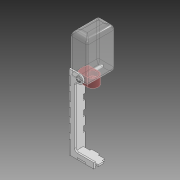
# Autodesk Inventor part: Узел_наклона
Saved by Autodesk Inventor 2022 (Build 260153000, 153)
## iProperties
Created: 2025-01-31
Part Number: Узел_наклона
Material: Типовые
Document SubType Name: Modeling
Designer: Ivan
Density: 1 g/cm^3
Appearance: По умолчанию
Author: Ivan
Autodesk Inventor part; units mm, degrees
ref_plane "YZ Plane" through (0, 0, 0) normal (1, 0, 0) x (0, 1, 0)
ref_plane "XZ Plane" through (0, 0, 0) normal (0, 1, 0) x (-1, 0, 0)
ref_plane "XY Plane" through (0, 0, 0) normal (0, 0, 1) x (1, 0, 0)
sketch "Эскиз1" plane through (0, 0, 0) normal (0, 0, 1) x (1, 0, 0)
  line L0 (0, 0) -> (0, 30.9191)
  line L1 (5, 0) -> (5, 15)
  line L2 (5, 15) -> (15.25, 15)
  line L3 (15.25, 15) -> (15.25, 31)
  line L4 (15.25, 31) -> (40, 31)
  line L5 (40, 31) -> (40, 0)
  line L6 (40, 0) -> (5, 0)
  dimension "d0" = 10
  dimension "d1" = 30.5
  dimension "d2" = 16
  dimension "d3" = 15
  dimension "d4" = 80
  constraints: 14 end point, 5 perpendicular, 2 vertical, 1 point on line
  measures "d0" diameter of L1 L0
  measures "d1" diameter of L3 L0
  measures "d2" distance of L2.end L3.end
  measures "d3" distance of L1.start L1.end
  measures "d4" diameter of L5 L0
revolve "Вращение1" add sketch "Эскиз1" angle 360 about axis through (0, 0, 0) along (0, 1, 0)
sketch "Эскиз2" plane through (0, 15, 0) normal (0, 1, 0) x (1, 0, 0)
  ellipse E0 centre (0, 0) end of major axis (0, 14) minor radius 8
  dimension "d6" = 14
  dimension "d7" = 8
  constraints: 1 coincident, 2 other
extrude "Выдавливание1" cut sketch "Эскиз2" against normal through all
sketch "Эскиз3" plane through (0, 0, 0) normal (0, 0, 1) x (1, 0, 0)
  circle A0 centre (-25, 15.5) radius 4.1
  line L0 (-40, 31) -> (-40, 0) construction
  point P0 (0, 0)
  point P1 (-40, 15.5)
  dimension "d10" = 8.2
  dimension "d11" = 25
  constraints: 1 centre point, 1 horizontal alignment, 1 midpoint
  measures "d10" diameter of A0
  measures "d11" horizontal distance of point (0, 0) A0.centre
extrude "Выдавливание2" cut sketch "Эскиз3" along normal through all both and the other way through all
sketch "Эскиз4" plane through (0, 31, 0) normal (0, 1, 0) x (1, 0, 0)
  line L0 (45.6039, -20) -> (-45.6039, -20)
  line L1 (-45.6039, -20) -> (-45.6039, 20)
  line L2 (-45.6039, 20) -> (45.6039, 20)
  line L3 (45.6039, 20) -> (45.6039, -20)
  ellipse E0 centre (0, 0) end of major axis (0, 14) minor radius 8 projected
  line L4 (45.6039, -20) -> (-45.6039, 20) construction
  line L5 (-45.6039, -20) -> (45.6039, 20) construction
  line L6 (-60.9114, -53.5893) -> (60.9114, -53.5893)
  line L7 (60.9114, -53.5893) -> (60.9114, 53.5893)
  line L8 (60.9114, 53.5893) -> (-60.9114, 53.5893)
  line L9 (-60.9114, 53.5893) -> (-60.9114, -53.5893)
  line L10 (-60.9114, -53.5893) -> (60.9114, 53.5893) construction
  line L11 (60.9114, -53.5893) -> (-60.9114, 53.5893) construction
  circle A0 centre (0, 0) radius 20
  point P0 (0, 20)
  point P1 (0, -20)
  dimension "d14" = 40
  constraints: 24 end point, 4 midpoint, 4 parallel, 2 horizontal, 2 perpendicular, 1 centre point, 1 coincident, 1 tangent, 1 other
  measures "d14" distance of L0.end L1.end
extrude "Выдавливание3" cut sketch "Эскиз4" against normal through all contours L0 A0 L2 L3 | L9 L8 L7 L6
fillet "Сопряжение1" radius 5 2 edges at (-34.641, 15.5, 20) (-34.641, 15.5, -20)
sketch "Эскиз5" plane through (0, 0, 0) normal (1, 0, 0) x (0, 1, 0)
  line L0 (0, 0) -> (47.7229, 0) construction
  line L1 (31, 17.1429) -> (31, -17.1429) projected
  line L2 (10.8203, 0) -> (31, 0)
  line L3 (31, 0) -> (31, -15.8105)
  line L4 (31, -15.8105) -> (10.8203, -15.8105)
  line L5 (10.8203, -15.8105) -> (10.8203, 0)
  constraints: 10 end point, 2 horizontal, 2 parallel, 2 point on line, 1 perpendicular
revolve "Вращение2" add sketch "Эскиз5" angle 360 about axis through (0, 0, 0) along (0, 1, 0) separate body
sketch "Эскиз6" plane through (0, 31, 0) normal (0, 1, 0) x (1, 0, 0)
  line L0 (25, 50) -> (-25, 50)
  line L1 (-30, 45) -> (-30, -45)
  line L2 (-25, -50) -> (25, -50)
  line L3 (30, -45) -> (30, 45)
  line L4 (30, 50) -> (-30, -50) construction
  line L5 (-30, 50) -> (30, -50) construction
  arc A0 (25, -50) -> (30, -45) centre (25, -45) ccw
  arc A1 (-30, -45) -> (-25, -50) centre (-25, -45) ccw
  arc A2 (-25, 50) -> (-30, 45) centre (-25, 45) ccw
  arc A3 (30, 45) -> (25, 50) centre (25, 45) ccw
  point P0 (0, 0)
  dimension "d19" = 100
  dimension "d20" = 60
  dimension "d21" = 5
  constraints: 12 end point, 8 point on circle, 8 point on line, 8 tangent, 4 centre point, 3 equal radius, 2 midpoint, 2 parallel, 1 horizontal, 1 perpendicular
  measures "d19" distance of L5.start L4.end
  measures "d20" distance of L4.end L5.end
  measures "d21" radius of A0
extrude "Выдавливание4" add sketch "Эскиз6" along normal blind 150 bodies 2
fillet "Сопряжение2" radius 20 8 edges at (-28.5355, 181, -48.5355) (-30, 181, 0) (-28.5355, 181, 48.5355) (0, 181, 50) (28.5355, 181, 48.5355) (30, 181, 0) (28.5355, 181, -48.5355) (0, 181, -50)
fillet "Сопряжение3" radius 10 8 edges at (-28.5355, 31, 48.5355) (0, 31, 50) (28.5355, 31, 48.5355) (30, 31, 0) (28.5355, 31, -48.5355) (0, 31, -50) (-28.5355, 31, -48.5355) (-30, 31, 0)
sketch "Эскиз7" plane through (0, 0, 0) normal (0, 0, 1) x (1, 0, 0)
  circle A0 centre (-25, 15.5) radius 4.1 projected
  point P0 (0, 0)
extrude "Выдавливание5" add sketch "Эскиз7" along normal blind 26 and the other way blind 60 separate body
sketch "Эскиз8" plane through (0, 0, 20) normal (0, 0, 1) x (1, 0, 0)
  circle A0 centre (-25, 15.5) radius 4.1 construction
  circle A1 centre (-25, 15.5) radius 4.1 construction
  circle A2 centre (-25, 15.5) radius 15.5
  line L0 (0, 31) -> (-31.6228, 31) construction
  line L1 (-10.4348, 20.8013) -> (30, -90.2923)
  line L2 (30, -90.2923) -> (30, -239)
  line L3 (-15.8105, 10.8203) -> (15.8105, 10.8203) construction
  line L4 (30, -239) -> (-60, -239)
  line L5 (-60, -239) -> (-60, 31)
  line L6 (-60, 31) -> (-25, 31)
  arc A3 (-30, 41) -> (-20, 31) centre (-20, 41) ccw projected
  line L7 (0, 0) -> (0, -302.6843) construction
  line L8 (-40, 31) -> (-40, 0) construction
  circle A4 centre (-25, 15.5) radius 10.9
  dimension "d30" = 270
  dimension "d31" = 20
  dimension "d32" = 20
  dimension "d33" = 90
  dimension "d34" = 21.8
  constraints: 12 end point, 3 perpendicular, 3 point on circle, 3 tangent, 2 centre point, 2 coincident, 1 horizontal, 1 vertical
  measures "d30" distance between parallel lines of L4 L6
  measures "d31" angle of L2 L1
  measures "d32" distance between parallel lines of L8 L5
  measures "d33" distance between parallel lines of L2 L5
  measures "d34" diameter of A4
extrude "Выдавливание6" add sketch "Эскиз8" along normal blind 6 separate body
sketch "Эскиз9" plane through (0, 0, 20) normal (0, 0, 1) x (1, 0, 0)
  circle A0 centre (-25, 15.5) radius 10.9 projected
  circle A1 centre (-25, 15.5) radius 4.1 projected
  point P0 (0, 0)
extrude "Выдавливание7" add sketch "Эскиз9" along normal blind 7 separate body
sketch "Эскиз10" plane through (-60, -239, 20) normal (-1, 0, 0) x (0, 0, 1)
  line L0 (6, 270) -> (-46, 270)
  line L1 (-46, 270) -> (-46, 0)
  line L2 (-46, 0) -> (6, 0)
  line L3 (6, 0) -> (6, 270)
  line L4 (-40, 270) -> (-40, 239) construction
  point P0 (-20, 239)
  dimension "d39" = 6
  constraints: 8 end point, 2 parallel, 1 horizontal, 1 perpendicular, 1 point on line
  measures "d39" distance between parallel lines of L1 L4
extrude "Выдавливание8" add sketch "Эскиз10" against normal blind 6 separate body
sketch "Эскиз11" plane through (-60, -239, 20) normal (0, -1, 0) x (1, 0, 0)
  line L0 (0, 6) -> (90, 6) projected
  line L1 (0, 6) -> (90, 6)
  line L2 (90, 6) -> (90, -46)
  line L3 (90, -46) -> (0, -46)
  line L4 (0, -46) -> (0, 6)
  line L5 (90, 0) -> (90, 6) projected
  line L6 (0, -46) -> (6, -46) projected
  point P0 (60, -20)
  constraints: 8 end point, 2 collinear, 2 parallel, 1 horizontal, 1 perpendicular
extrude "Выдавливание9" add sketch "Эскиз11" against normal blind 6 separate body
sketch "Эскиз12" plane through (-60, -239, 20) normal (-1, 0, 0) x (0, 0, 1)
  line L0 (-20, 239) -> (-20, 10.9172) construction
  line L1 (-46, 0) -> (-46, 270) construction
  line L2 (-46, 135) -> (6, 135) construction
  line L3 (6, 270) -> (6, 0) construction
  line L4 (6, 0) -> (-46, 0) construction
  line L5 (-30, 0) -> (-10, 0)
  line L6 (-10, 0) -> (-10, 6)
  line L7 (-10, 6) -> (-30, 6)
  line L8 (-30, 6) -> (-30, 0)
  line L9 (6, 120) -> (0, 120)
  line L10 (0, 120) -> (0, 100)
  line L11 (0, 100) -> (6, 100)
  line L12 (6, 100) -> (6, 120)
  line L13 (6, 70) -> (0, 70)
  line L14 (0, 70) -> (0, 50)
  line L15 (0, 50) -> (6, 50)
  line L16 (6, 50) -> (6, 70)
  line L17 (6, 150) -> (0, 150)
  line L18 (0, 150) -> (0, 170)
  line L19 (0, 170) -> (6, 170)
  line L20 (6, 170) -> (6, 150)
  line L21 (6, 200) -> (0, 200)
  line L22 (0, 200) -> (0, 220)
  line L23 (0, 220) -> (6, 220)
  line L24 (6, 220) -> (6, 200)
  line L25 (-46, 120) -> (-40, 120)
  line L26 (-40, 120) -> (-40, 100)
  line L27 (-40, 100) -> (-46, 100)
  line L28 (-46, 100) -> (-46, 120)
  line L29 (-46, 70) -> (-40, 70)
  line L30 (-40, 70) -> (-40, 50)
  line L31 (-40, 50) -> (-46, 50)
  line L32 (-46, 50) -> (-46, 70)
  line L33 (-40, 150) -> (-40, 170)
  line L34 (-40, 170) -> (-46, 170)
  line L35 (-46, 170) -> (-46, 150)
  line L36 (-46, 200) -> (-40, 200)
  line L37 (-40, 200) -> (-40, 220)
  line L38 (-40, 220) -> (-46, 220)
  line L39 (-46, 220) -> (-46, 200)
  line L40 (-46, 150) -> (-40, 150)
  line L41 (6, 148.7077) -> (6, 259.8013) projected
  line L42 (6, 250) -> (0, 250)
  line L43 (0, 250) -> (0, 270)
  line L44 (0, 270) -> (6, 270)
  line L45 (6, 270) -> (6, 250)
  line L46 (0, 270) -> (6, 270) projected
  line L47 (-46, 250) -> (-40, 250)
  line L48 (-40, 250) -> (-40, 270)
  line L49 (-40, 270) -> (-46, 270)
  line L50 (-46, 270) -> (-46, 250)
  line L51 (-40, 270) -> (-46, 270)
  point P0 (-46, 259.8013)
  dimension "d44" = 6
  dimension "d45" = 20
  dimension "d46" = 20
  dimension "d47" = 6
  dimension "d48" = 15
  dimension "d49" = 30
  constraints: 94 end point, 31 symmetric about line, 8 parallel, 8 point on line, 4 horizontal, 4 perpendicular, 3 equal length, 2 midpoint, 1 collinear, 1 vertical, 1 other
  measures "d44" distance of L5.end L6.end
  measures "d45" distance of L6.end L7.end
  measures "d46" distance of L9.end L10.end
  measures "d47" distance of L9.start L9.end
  measures "d48" distance between parallel lines of L2 L9
  measures "d49" distance between parallel lines of L13 L11
extrude "Выдавливание10" cut sketch "Эскиз12" against normal through all bodies 6
sketch "Эскиз13" plane through (0, 0, 26) normal (0, 0, 1) x (1, 0, 0)
  line L0 (-60, -19) -> (-54, -19) projected
  line L1 (-54, -89) -> (-54, -119) projected
  line L2 (-60, -239) -> (-60, -189) projected
  line L3 (-60, -69) -> (-54, -69) projected
  line L4 (-54, -39) -> (-54, -69)
  line L5 (-54, -39) -> (-60, -39) projected
  line L6 (-60, -69) -> (-60, -39) projected
  line L7 (-54, -89) -> (-60, -89) projected
  line L8 (-60, -119) -> (-60, -89)
  line L9 (-60, -119) -> (-54, -119) projected
  line L10 (-54, -89) -> (-54, -119) projected
  line L11 (-60, -169) -> (-54, -169) projected
  line L12 (-54, -139) -> (-54, -169) projected
  line L13 (-54, -139) -> (-60, -139) projected
  line L14 (-60, -169) -> (-60, -139)
  line L15 (-54, -189) -> (-60, -189) projected
  line L16 (-60, -239) -> (-60, -189) projected
  line L17 (-60, -239) -> (-54, -239) projected
  line L18 (-54, -189) -> (-54, -239)
  line L19 (-60, -239) -> (30, -239) construction
  line L20 (-30, -239) -> (0, -239)
  line L21 (0, -239) -> (0, -233)
  line L22 (0, -233) -> (-30, -233)
  line L23 (-30, -233) -> (-30, -239)
  line L24 (-60, -119) -> (-54, -119) projected
  line L25 (-54, -89) -> (-60, -89) projected
  line L26 (-60, -119) -> (-60, -89) projected
  line L27 (-54, -139) -> (-60, -139) projected
  line L28 (-60, -169) -> (-60, -139) projected
  line L29 (-60, -169) -> (-54, -169) projected
  line L30 (-54, -139) -> (-54, -169) projected
  line L31 (-54, 11) -> (-54, -19)
  line L32 (-54, 11) -> (-60, 11) projected
  line L33 (-60, -19) -> (-60, 11) projected
  line L34 (-54, -39) -> (-60, -39) projected
  line L35 (-60, -69) -> (-60, -39) projected
  line L36 (-60, -69) -> (-54, -69) projected
  line L37 (-54, -39) -> (-54, -69) projected
  line L38 (-54, -189) -> (-60, -189) projected
  line L39 (-60, -239) -> (-54, -239) projected
  line L40 (-54, -189) -> (-54, -239) projected
  point P0 (0, 0)
  point P1 (-15, -239)
  point P2 (-15, -239)
  dimension "d52" = 30
  constraints: 18 end point, 2 midpoint, 2 parallel, 2 perpendicular, 1 coincident, 1 horizontal, 1 point on line
  measures "d52" distance of L21.end L22.end
extrude "Выдавливание11" cut sketch "Эскиз13" against normal through all bodies 4
sketch "Эскиз14" plane through (-60, -239, 20) normal (0, -1, 0) x (1, 0, 0)
  line L0 (90, -46) -> (0, -46) construction
  line L1 (45, -46) -> (45, 5.2273) construction
  line L2 (45.9, 7) -> (24.1, 7) construction
  line L3 (60, -20) -> (-12.0098, -20) construction
  line L4 (0, -10) -> (6, -10) projected
  line L5 (6, 6) -> (6, -10) projected
  line L6 (0, 6) -> (6, 6) projected
  line L7 (0, -10) -> (0, 6) projected
  line L8 (6, -30) -> (0, -30) projected
  line L9 (0, -46) -> (0, -30) projected
  line L10 (0, -46) -> (6, -46) projected
  line L11 (6, -30) -> (6, -46) projected
  line L12 (6, 6) -> (6, 0) projected
  line L13 (60, 0) -> (90, 0) projected
  line L14 (30, 0) -> (30, 6) projected
  line L15 (6, 6) -> (30, 6) projected
  line L16 (60, 6) -> (60, 0) projected
  line L17 (60, 0) -> (90, 0) projected
  line L18 (90, 0) -> (90, 6) projected
  line L19 (60, 6) -> (90, 6)
  line L20 (90, -10) -> (84, -10)
  line L21 (84, 6) -> (84, -10)
  line L22 (90, 6) -> (84, 6)
  line L23 (90, -10) -> (90, 6)
  line L24 (84, -30) -> (90, -30)
  line L25 (90, -46) -> (90, -30)
  line L26 (90, -46) -> (84, -46)
  line L27 (84, -30) -> (84, -46)
  line L28 (84, 6) -> (84, 0)
  line L29 (45.9, -47) -> (24.1, -47) construction
  line L30 (0, -46) -> (6, -46)
  line L31 (6, -46) -> (6, -40)
  line L32 (6, -40) -> (30, -40)
  line L33 (30, -40) -> (30, -46)
  line L34 (6, -46) -> (30, -46)
  line L35 (60, -46) -> (60, -40)
  line L36 (60, -40) -> (90, -40)
  line L37 (90, -40) -> (90, -46)
  line L38 (60, -46) -> (90, -46)
  line L39 (84, -46) -> (84, -40)
  line L40 (90, -46) -> (84, -46)
  line L41 (6, 0) -> (30, 0)
  line L42 (60, 6) -> (60, 0) projected
  line L43 (90, 0) -> (90, 6) projected
  line L44 (60, 6) -> (90, 6) projected
  point P0 (102.0098, -20)
  point P1 (45, -45.2273)
  constraints: 50 end point, 25 symmetric about line, 1 horizontal, 1 midpoint, 1 perpendicular
extrude "Выдавливание12" cut sketch "Эскиз14" against normal through all bodies 7
sketch "Эскиз15" plane through (0, 0, 26) normal (0, 0, 1) x (1, 0, 0)
  circle A0 centre (-25, 15.5) radius 4.1 projected
  circle A1 centre (-25, 15.5) radius 4.1 projected
  arc A2 (-10.4348, 20.8013) -> (-25, 31) centre (-25, 15.5) ccw projected
  circle A3 centre (-25, 15.5) radius 15.5
  line L0 (-31.6228, 0) -> (0, 0) projected
  line L1 (-40, -219) -> (30, -219)
  line L2 (30, -239) -> (30, -90.2923) projected
  line L3 (30, -90.2923) -> (-10.4348, 20.8013) projected
  line L4 (0, -239) -> (30, -239) projected
  line L5 (-25, 0) -> (-40, 0)
  line L6 (-40, 0) -> (-40, -219)
  point P0 (-10.4348, 20.8013)
  dimension "d59" = 20
  dimension "d63" = 70
  constraints: 6 end point, 2 horizontal, 2 point on circle, 2 point on line, 1 centre point, 1 coincident, 1 perpendicular
  measures "d59" distance between parallel lines of L4 L1
  measures "d63" distance between parallel lines of L6 L2
extrude "Выдавливание13" cut sketch "Эскиз15" against normal through all contours L3 L0 A3 | L3 L2 L1 L6 L5 L0 bodies 4
fillet "Сопряжение4" radius 10 3 edges at (-25, 0, 23) (-40, 0, 23) (-40, -219, 23)
sketch "Эскиз16" plane through (-60, -239, 20) normal (-1, 0, 0) x (0, 0, 1)
  line L0 (-37.1429, 270) -> (-2.8571, 270) construction
  line L1 (-40, 270) -> (0, 270)
  line L2 (0, 270) -> (0, 238)
  line L3 (0, 238) -> (-40, 238)
  line L4 (-40, 238) -> (-40, 270)
  point P0 (-20, 239)
  point P1 (-20, 270)
  point P2 (-20, 270)
  dimension "d64" = 40
  dimension "d65" = 32
  constraints: 8 end point, 2 midpoint, 2 parallel, 1 coincident, 1 horizontal, 1 perpendicular, 1 point on line
  measures "d64" distance of L2.end L3.end
  measures "d65" distance of L1.end L2.end
extrude "Выдавливание14" cut sketch "Эскиз16" against normal through all bodies 6
equation "\"d46\" = d45"
equation "\"d47\" = d44"
equation "\"d48\" = 0.5 * d49"
